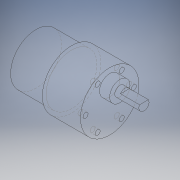
# Autodesk Inventor part: Nextrox-Mini-12VDC-60rpmGearbox-Motor
Saved by Autodesk Inventor 2017 (Build 210142000, 142)
## iProperties
Created: 2018-04-08
Part Number: Nextrox-Mini-12VDC-60rpmGearbox-Motor
Material: Stainless Steel
Document SubType Name: Modeling
Designer: MtgSaber
Density: 8 g/cm^3
Appearance: Semi-Polished
Author: MtgSaber
Autodesk Inventor part; units mm, degrees
ref_plane "YZ Plane" through (0, 0, 0) normal (1, 0, 0) x (0, 1, 0)
ref_plane "XZ Plane" through (0, 0, 0) normal (0, 1, 0) x (-1, 0, 0)
ref_plane "XY Plane" through (0, 0, 0) normal (0, 0, 1) x (1, 0, 0)
sketch "Sketch1" plane through (0, 0, 0) normal (1, 0, 0) x (0, 1, 0)
  circle A0 centre (0, 0) radius 15.875
  dimension "d0" = 31.75
  constraints: 1 centre point, 1 coincident
  measures "d0" diameter of A0
extrude "Extrusion1" add sketch "Sketch1" along normal blind 22.225
sketch "Sketch2" plane through (22.225, 0, 0) normal (1, 0, 0) x (0, 0, -1)
  circle A0 centre (0, 0) radius 15.875 construction
  circle A1 centre (0, 0) radius 18.2563
  dimension "d3" = 36.5125
  constraints: 1 centre point, 1 coincident
  measures "d3" diameter of A1
extrude "Extrusion2" add sketch "Sketch2" along normal blind 23.8125
sketch "Sketch3" plane through (46.0375, 0, 0) normal (1, 0, 0) x (0, 0, -1)
  circle A0 centre (0, 8.7313) radius 6.35
  circle A1 centre (0, 8.7313) radius 8.7313 construction
  line L0 (0, -25.5588) -> (0, 25.5588) construction
  point P0 (0, 0)
  dimension "d13" = 17.4625
  dimension "d7" = 12.7
  constraints: 1 centre point, 1 coincident, 1 point on line, 1 vertical alignment, 2 other
  measures "d7" diameter of A0
extrude "Extrusion3" add sketch "Sketch3" along normal blind 6.35
sketch "Sketch4" plane through (52.3875, 8.7313, 0) normal (1, 0, 0) x (0, 0, -1)
  circle A0 centre (0, 0) radius 3.175
  circle A1 centre (0, 0) radius 6.35 construction
  point P0 (0, -8.7313)
  dimension "d10" = 6.35
  constraints: 1 centre point, 1 concentric
  measures "d10" diameter of A0
extrude "Extrusion4" add sketch "Sketch4" along normal blind 15.0812
sketch "Sketch5" plane through (46.0375, 0, 0) normal (1, 0, 0) x (0, 0, -1)
  circle A0 centre (0, 0) radius 15.0812 construction
  line L0 (25.5588, 0) -> (-25.5588, 0) construction
  point P0 (15.0812, 0)
  dimension "d14" = 30.1625
  constraints: 1 coincident, 1 horizontal alignment, 1 point on line, 2 other
hole "Hole1" at (46.0375, 0, -15.0812) direction (-1, 0, 0) diameter 3.175 depth 3.175
pattern_circular "Circular Pattern1" count 6 over 360 about axis through (-10, 0, 0) along (1, 0, 0) of "Hole1"
sketch "Sketch6" plane through (67.4687, 8.7313, 0) normal (1, 0, 0) x (0, 0, -1)
  circle A0 centre (0, 0) radius 3.175 construction
  line L0 (-2.7781, 1.5371) -> (2.7781, 1.5371)
  arc A1 (2.7781, 1.5371) -> (-2.7781, 1.5371) centre (0, 0) ccw
  point P0 (0, -8.7313)
  dimension "d25" = 5.5563
  constraints: 4 point on circle, 2 end point, 1 centre point, 1 coincident, 1 horizontal
  measures "d25" distance of L0.start L0.end
extrude "Extrusion5" cut sketch "Sketch6" against normal blind 11.9062
body "Solid1"
